Autodesk Inventor part; units mm, degrees
(part 2 of 2)
  spline S168 degree 2 poles (-46.712, 7.0194) (-46.712, 7.138) (-46.7021, 7.2566) (-46.6873, 7.3308) knots 0 0 0 1 2 2 2
  line L186 (-46.6873, 7.3308) -> (-45.8865, 7.3308)
  line L187 (-42.1345, 8.7149) -> (-42.1345, 7.9438)
  line L188 (-42.1345, 7.9438) -> (-46.712, 7.9438)
  line L189 (-46.712, 7.9438) -> (-46.712, 8.7149)
  line L190 (-46.712, 8.7149) -> (-42.1345, 8.7149)
  line L191 (-47.4732, 8.7693) -> (-47.4732, 7.8943)
  line L192 (-47.4732, 7.8943) -> (-48.2741, 7.8943)
  line L193 (-48.2741, 7.8943) -> (-48.2741, 8.7693)
  line L194 (-48.2741, 8.7693) -> (-47.4732, 8.7693)
  line L195 (-42.1345, 13.4011) -> (-42.1345, 12.457)
  line L196 (-42.1345, 12.457) -> (-43.8548, 11.3447)
  line L197 (-43.8548, 11.3447) -> (-42.1345, 10.2028)
  line L198 (-42.1345, 10.2028) -> (-42.1345, 9.3279)
  line L199 (-42.1345, 9.3279) -> (-44.4035, 10.9147)
  line L200 (-44.4035, 10.9147) -> (-46.712, 9.3427)
  line L201 (-46.712, 9.3427) -> (-46.712, 10.2869)
  line L202 (-46.712, 10.2869) -> (-45.0065, 11.3942)
  line L203 (-45.0065, 11.3942) -> (-46.712, 12.5262)
  line L204 (-46.712, 12.5262) -> (-46.712, 13.4011)
  line L205 (-46.712, 13.4011) -> (-44.4529, 11.8242)
  line L206 (-44.4529, 11.8242) -> (-42.1345, 13.4011)
  line L207 (-44.2305, 20.4305) -> (-44.2305, 19.7038)
  line L208 (-44.2305, 19.7038) -> (-42.1345, 19.7038)
  line L209 (-42.1345, 19.7038) -> (-42.1345, 18.9178)
  line L210 (-42.1345, 18.9178) -> (-44.2305, 18.9178)
  line L211 (-44.2305, 18.9178) -> (-44.2305, 16.2237)
  line L212 (-44.2305, 16.2237) -> (-45.0906, 16.2237)
  line L213 (-45.0906, 16.2237) -> (-48.2345, 18.9524)
  line L214 (-48.2345, 18.9524) -> (-48.2345, 19.7038)
  line L215 (-48.2345, 19.7038) -> (-44.8879, 19.7038)
  line L216 (-44.8879, 19.7038) -> (-44.8879, 20.4305)
  line L217 (-44.8879, 20.4305) -> (-44.2305, 20.4305)
  line L218 (-44.8879, 18.9178) -> (-47.2706, 18.9178)
  line L219 (-47.2706, 18.9178) -> (-44.8879, 16.8664)
  line L220 (-44.8879, 16.8664) -> (-44.8879, 18.9178)
  line L221 (-42.1345, 24.7509) -> (-42.1345, 23.8067)
  line L222 (-42.1345, 23.8067) -> (-43.8548, 22.6945)
  line L223 (-43.8548, 22.6945) -> (-42.1345, 21.5526)
  line L224 (-42.1345, 21.5526) -> (-42.1345, 20.6776)
  line L225 (-42.1345, 20.6776) -> (-44.4035, 22.2644)
  line L226 (-44.4035, 22.2644) -> (-46.712, 20.6925)
  line L227 (-46.712, 20.6925) -> (-46.712, 21.6366)
  line L228 (-46.712, 21.6366) -> (-45.0065, 22.7439)
  line L229 (-45.0065, 22.7439) -> (-46.712, 23.8759)
  line L230 (-46.712, 23.8759) -> (-46.712, 24.7509)
  line L231 (-46.712, 24.7509) -> (-44.4529, 23.174)
  line L232 (-44.4529, 23.174) -> (-42.1345, 24.7509)
  line L233 (-44.2305, 29.1603) -> (-44.2305, 28.4336)
  line L234 (-44.2305, 28.4336) -> (-42.1345, 28.4336)
  line L235 (-42.1345, 28.4336) -> (-42.1345, 27.6476)
  line L236 (-42.1345, 27.6476) -> (-44.2305, 27.6476)
  line L237 (-44.2305, 27.6476) -> (-44.2305, 24.9536)
  line L238 (-44.2305, 24.9536) -> (-45.0906, 24.9536)
  line L239 (-45.0906, 24.9536) -> (-48.2345, 27.6822)
  line L240 (-48.2345, 27.6822) -> (-48.2345, 28.4336)
  line L241 (-48.2345, 28.4336) -> (-44.8879, 28.4336)
  line L242 (-44.8879, 28.4336) -> (-44.8879, 29.1603)
  line L243 (-44.8879, 29.1603) -> (-44.2305, 29.1603)
  line L244 (-44.8879, 27.6476) -> (-47.2706, 27.6476)
  line L245 (-47.2706, 27.6476) -> (-44.8879, 25.5962)
  line L246 (-44.8879, 25.5962) -> (-44.8879, 27.6476)
  point P0 (0, 0)
  constraints: 2 other
extrude "Extrusion5" cut sketch "Sketch5" against normal blind 0.5
body "Solid1"
